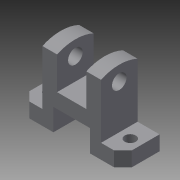
# Autodesk Inventor part: HW 5 Part 2
Saved by Autodesk Inventor 2015 SP1 (Build 190203100, 203)
## iProperties
Created: 2016-02-03
Part Number: HW 5 Part 2
Material: Generic
Document SubType Name: Modeling
Designer: melissa.roth
Density: 1 g/cm^3
Appearance: Default
Author: melissa.roth
Autodesk Inventor part; units mm, degrees
ref_plane "YZ Plane" through (0, 0, 0) normal (1, 0, 0) x (0, 1, 0)
ref_plane "XZ Plane" through (0, 0, 0) normal (0, 1, 0) x (-1, 0, 0)
ref_plane "XY Plane" through (0, 0, 0) normal (0, 0, 1) x (1, 0, 0)
sketch "Sketch1" plane through (0, 0, 0) normal (0, 0, 1) x (1, 0, 0)
  line L0 (0, 0) -> (28.575, 0)
  line L1 (28.575, 0) -> (28.575, 19.05)
  line L2 (28.575, 19.05) -> (60.325, 19.05)
  line L3 (60.325, 19.05) -> (60.325, 0)
  line L4 (60.325, 0) -> (88.9, 0)
  line L5 (88.9, 0) -> (88.9, 12.7)
  line L6 (88.9, 12.7) -> (69.85, 12.7)
  line L7 (69.85, 12.7) -> (69.85, 63.5)
  line L8 (69.85, 63.5) -> (57.15, 63.5)
  line L9 (57.15, 63.5) -> (57.15, 31.75)
  line L10 (57.15, 31.75) -> (31.75, 31.75)
  line L11 (31.75, 31.75) -> (31.75, 63.5)
  line L12 (31.75, 63.5) -> (19.05, 63.5)
  line L13 (19.05, 63.5) -> (19.05, 12.7)
  line L14 (19.05, 12.7) -> (0, 12.7)
  line L15 (0, 12.7) -> (0, 0)
  dimension "d0" = 19.05
  dimension "d1" = 31.75
  dimension "d2" = 12.7
  dimension "d3" = 25.4
  dimension "d4" = 88.9
  dimension "d5" = 50.8
  dimension "d6" = 19.05
  dimension "d7" = 12.7
  constraints: 32 end point, 13 perpendicular, 4 equal length, 4 point on line, 1 horizontal
  measures "d0" distance of L0.end L1.end
  measures "d1" distance of L1.end L2.end
  measures "d2" distance of L4.end L5.end
  measures "d3" distance between parallel lines of L9 L11
  measures "d4" distance of L5.end L14.end
  measures "d5" distance of L6.end L7.end
  measures "d6" distance of L13.end L14.end
  measures "d7" distance between parallel lines of L10 L2
extrude "Extrusion1" add sketch "Sketch1" along normal blind 31.75
sketch "Sketch2" plane through (69.85, 12.7, 0) normal (1, 0, 0) x (0, 0, -1)
  point P0 (0, -12.7)
sketch "Sketch3" plane through (69.85, 12.7, 0) normal (1, 0, 0) x (0, 0, -1)
  point P0 (0, -12.7)
sketch "Sketch4" plane through (69.85, 12.7, 0) normal (1, 0, 0) x (0, 0, -1)
  line L0 (0, 0) -> (0, 50.8) projected
  line L1 (-31.75, 0) -> (-31.75, 50.8) projected
  arc A0 (0, 47.3352) -> (-31.75, 47.3352) centre (-15.875, 12.7) ccw
  line L2 (0, 50.8) -> (-31.75, 50.8) projected
  line L3 (-31.75, 47.3352) -> (-31.75, 51.0727)
  line L4 (-31.75, 51.0727) -> (0, 51.0727)
  line L5 (0, 51.0727) -> (0, 47.3352)
  point P0 (0, -12.7)
  dimension "d10" = 38.1
  constraints: 6 end point, 2 perpendicular, 2 point on circle, 2 point on line, 1 centre point, 1 tangent, 1 vertical
  measures "d10" radius of A0
extrude "Extrusion2" cut sketch "Sketch4" against normal through all
sketch "Sketch5" plane through (69.85, 12.7, 31.75) normal (1, 0, 0) x (0, 0, -1)
  circle A0 centre (15.875, 38.1) radius 6.35
  line L0 (31.75, 0) -> (31.75, 47.3352) projected
  line L1 (31.75, 0) -> (0, 0) projected
  point P0 (31.75, -12.7)
  dimension "d13" = 12.7
  dimension "d14" = 15.875
  dimension "d15" = 38.1
  constraints: 1 centre point
  measures "d13" diameter of A0
  measures "d14" distance from line of L0 A0.centre
  measures "d15" distance from line of L1 A0.centre
extrude "Extrusion3" cut sketch "Sketch5" against normal through all
chamfer "Chamfer1" distance 7.62 angle 45 1 edges at (88.9, 6.35, 31.75)
chamfer "Chamfer2" distance 7.62 angle 45 1 edges at (0, 6.35, 31.75)
sketch "Sketch7" plane through (69.85, 12.7, 0) normal (0, 1, 0) x (1, 0, 0)
  circle A0 centre (9.525, -15.875) radius 4.7625
  circle A1 centre (-60.325, -15.875) radius 4.7625
  line L0 (19.05, 0) -> (0, 0) projected
  line L1 (19.05, 0) -> (19.05, -24.13) projected
  line L2 (-50.8, 0) -> (-69.85, 0) projected
  line L3 (-69.85, 0) -> (-69.85, -24.13) projected
  dimension "d24" = 9.525
  dimension "d25" = 9.525
  dimension "d26" = 15.875
  dimension "d27" = 9.525
  dimension "d28" = 15.875
  dimension "d29" = 9.525
  constraints: 2 centre point
  measures "d24" diameter of A0
  measures "d25" diameter of A1
  measures "d26" distance from line of L0 A0.centre
  measures "d27" distance from line of L1 A0.centre
  measures "d28" distance from line of L2 A1.centre
  measures "d29" distance from line of L3 A1.centre
extrude "Extrusion4" cut sketch "Sketch7" against normal through all
equation "\"d0\" = 0.75 * d3"
equation "\"d1\" = 1.25 * d3"
equation "\"d2\" = 0.5 * d3"
equation "\"d4\" = 3.5 * d3"
equation "\"d5\" = 2 * d3"
equation "\"d6\" = 0.75 * d3"
equation "\"d7\" = 0.5 * d3"
equation "\"d25\" = d24"
equation "\"d28\" = d26"
equation "\"d29\" = d27"
body "Solid1"
